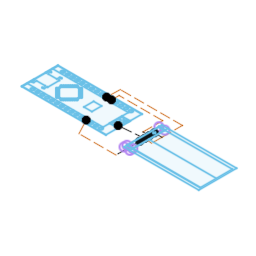
2020_09_18_Arduino & Bluetooth Wood Adaptator V2 v3 (Autodesk Fusion 360 design; units mm, degrees)
Autodesk Fusion 360 part; units mm, degrees
sketch "HC06" plane through (0, 0, 0) normal (0, 0, 1) x (1, 0, 0)
  line L0 (11.524, -5.694) -> (11.524, -4.694)
  line L1 (12.0236, -5.2144) -> (11.0244, -5.2144)
  line L2 (13.0183, 0.206) -> (9.8997, 0.206)
  line L3 (10.024, -1.294) -> (11.524, -1.294)
  circle A0 centre (11.524, -12.694) radius 0.5
  line L4 (10.024, -1.294) -> (11.524, -1.294)
  line L5 (47.724, -17.744) -> (10.024, -17.744)
  line L6 (47.724, -1.294) -> (10.024, -1.294)
  circle A1 centre (11.524, -12.694) radius 0.5
  line L7 (47.724, -9.519) -> (13.024, -9.519)
  line L8 (13.0199, -19.244) -> (48.4034, -19.244)
  line L9 (10.024, -1.294) -> (10.024, 0.206)
  line L10 (48.4034, -19.244) -> (48.4034, 0.206)
  line L11 (13.024, -17.744) -> (13.024, -19.244)
  line L12 (48.4034, 0.206) -> (13.0183, 0.206)
  line L13 (13.024, -1.294) -> (13.024, -17.744)
  line L14 (47.724, -17.744) -> (10.024, -17.744)
  line L15 (13.024, -1.294) -> (13.024, 0.206)
  circle A2 centre (11.524, -5.194) radius 0.5
  line L16 (10.024, -1.294) -> (13.024, -1.294)
  line L17 (47.724, -1.294) -> (47.724, -17.744)
  circle A3 centre (11.524, -5.194) radius 0.5
  line L18 (10.024, -17.744) -> (10.024, -1.294)
  circle A4 centre (11.524, -7.694) radius 0.5
  circle A5 centre (11.524, -7.694) radius 0.5
  line L19 (10.024, -1.294) -> (13.024, -1.294)
  circle A6 centre (11.524, -10.194) radius 0.5
  circle A7 centre (11.524, -10.194) radius 0.5
  line L20 (12.0236, -5.2144) -> (11.0244, -5.2144)
  line L21 (11.524, -5.694) -> (11.524, -4.694)
  line L22 (13.024, -1.294) -> (13.024, -17.744)
  line L23 (13.024, -19.244) -> (10.024, -19.244)
  line L24 (10.024, -17.744) -> (10.024, -1.294)
  line L25 (10.024, -17.744) -> (10.024, -19.244)
sketch "ArduinoNano" plane through (0, 0, 0) normal (0, 0, 1) x (1, 0, 0)
  arc A0 (-42.68, -4.5943) -> (-42.08, -4.5943) centre (-42.38, -4.2943) ccw
  line L0 (0, 0) -> (-43.18, 0)
  line L1 (-42.88, -12.271) -> (-43.18, -12.271)
  line L2 (-36.48, -13.7477) -> (-36.68, -13.9477)
  arc A1 (-36.68, -13.9477) -> (-37.28, -13.9477) centre (-36.98, -14.2477) ccw
  line L3 (-43.18, -6.271) -> (-42.88, -6.271)
  arc A2 (-37.28, -4.5943) -> (-36.68, -4.5943) centre (-36.98, -4.2943) ccw
  line L4 (0, -6.771) -> (0, 0)
  line L5 (-36.68, -4.5943) -> (-36.48, -4.7943)
  line L6 (-43.18, -18.542) -> (0, -18.542)
  line L7 (0, -11.771) -> (0, -6.771)
  arc A3 (-42.88, -13.7477) -> (-42.88, -12.271) centre (-43.6183, -13.0093) ccw
  line L8 (-42.88, -6.271) -> (-42.88, -4.7943)
  line L9 (-36.48, -6.271) -> (-36.18, -6.271)
  line L10 (-42.68, -13.9477) -> (-42.88, -13.7477)
  line L11 (-41.88, -6.271) -> (-37.48, -6.271)
  line L12 (-43.18, 0) -> (-43.18, -6.271)
  line L13 (-37.48, -4.7943) -> (-37.28, -4.5943)
  line L14 (-42.08, -4.5943) -> (-41.88, -4.7943)
  arc A4 (-37.48, -13.7477) -> (-37.48, -12.271) centre (-38.2183, -13.0093) ccw
  line L15 (-42.88, -4.7943) -> (-42.68, -4.5943)
  line L16 (-37.28, -13.9477) -> (-37.48, -13.7477)
  line L17 (-36.48, -12.271) -> (-36.48, -13.7477)
  line L18 (0, -18.542) -> (0, -11.771)
  arc A5 (-36.48, -4.7943) -> (-36.48, -6.271) centre (-35.7416, -5.5326) ccw
  line L19 (-36.18, -12.271) -> (-36.48, -12.271)
  line L20 (-37.48, -12.271) -> (-41.88, -12.271)
  line L21 (-37.48, -6.271) -> (-37.48, -4.7943)
  line L22 (-41.88, -12.271) -> (-41.88, -13.7477)
  line L23 (-36.18, -6.271) -> (-36.18, -12.271)
  arc A6 (-41.88, -4.7943) -> (-41.88, -6.271) centre (-41.1416, -5.5326) ccw
  circle A7 centre (-14.156, -1.524) radius 0.889
  circle A8 centre (-3, -9.271) radius 0.76
  arc A9 (-24.6374, -12.0012) -> (-24.6374, -12.2841) centre (-24.7789, -12.1427) cw
  arc A10 (-31.1356, -5.671) -> (-30.8528, -5.671) centre (-30.9942, -5.8124) cw
  line L24 (-25.3179, -11.9006) -> (-25.028, -11.6107)
  circle A11 centre (-14.156, -17.018) radius 0.889
  circle A12 centre (-3.0017, -7.271) radius 0.76
  line L25 (-18.0694, -11.771) -> (-18.0694, -6.771)
  line L26 (-18.0694, -6.771) -> (-13.9686, -6.771)
  circle A13 centre (-14.156, -17.018) radius 0.5
  circle A14 centre (-24.156, -1.524) radius 0.5
  circle A15 centre (-6.656, -17.018) radius 0.889
  line L27 (0, -6.0786) -> (0, -12.4635)
  circle A16 centre (-19.156, -17.018) radius 0.5
  line L28 (-4.2, -15.829) -> (-4.2, -2.8014)
  line L29 (-13.9686, -6.771) -> (-13.9686, -11.771)
  circle A17 centre (-11.656, -17.018) radius 0.889
  line L30 (-30.8528, -5.671) -> (-30.4622, -6.0616)
  line L31 (-30.7521, -6.3515) -> (-31.1427, -5.9609)
  line L32 (-4.2, -12.4635) -> (-4.2, -6.0786)
  circle A18 centre (-9.156, -1.524) radius 0.889
  circle A19 centre (-16.656, -1.524) radius 0.889
  line L33 (-31.1427, -5.6781) -> (-31.1356, -5.671)
  line L34 (-43.18, 0) -> (-43.18, -18.542)
  arc A20 (-42.08, -13.9477) -> (-42.68, -13.9477) centre (-42.38, -14.2477) ccw
  arc A21 (-31.2001, -12.8065) -> (-31.2001, -12.5236) centre (-31.0587, -12.665) cw
  line L35 (-13.9686, -11.771) -> (-18.0694, -11.771)
  line L36 (0, -12.4635) -> (-4.2, -12.4635)
  circle A22 centre (-9.156, -17.018) radius 0.5
  line L37 (-19.156, -1.524) -> (-19.156, -1.024)
  circle A23 centre (-6.656, -17.018) radius 0.5
  circle A24 centre (-16.656, -17.018) radius 0.889
  circle A25 centre (-19.156, -1.524) radius 0.5
  line L38 (-21.656, -1.524) -> (-21.656, -1.024)
  line L39 (-31.1931, -12.8135) -> (-31.2001, -12.8065)
  circle A26 centre (-6.656, -1.524) radius 0.5
  line L40 (-41.88, -13.7477) -> (-42.08, -13.9477)
  circle A27 centre (-9.156, -17.018) radius 0.889
  line L41 (-0.9965, -7.771) -> (-0.9965, -6.511)
  arc A28 (-24.6445, -12.2912) -> (-24.9274, -12.2912) centre (-24.7859, -12.1497) cw
  line L42 (-24.6374, -12.2841) -> (-24.6445, -12.2912)
  circle A29 centre (-14.156, -1.524) radius 0.5
  line L43 (-24.9274, -12.2912) -> (-25.3179, -11.9006)
  line L44 (-31.2001, -12.5236) -> (-30.8096, -12.133)
  line L45 (-30.4622, -6.0616) -> (-30.7521, -6.3515)
  arc A30 (-31.1427, -5.9609) -> (-31.1427, -5.6781) centre (-31.0013, -5.8195) cw
  line L46 (-19.156, -16.518) -> (-19.156, -17.018)
  circle A31 centre (-9.156, -1.524) radius 0.5
  arc A32 (-30.9102, -12.8135) -> (-31.1931, -12.8135) centre (-31.0517, -12.6721) cw
  line L47 (-24.156, -1.524) -> (-24.156, -1.024)
  line L48 (-12.156, -17.018) -> (-11.156, -17.018)
  circle A33 centre (-11.656, -1.524) radius 0.5
  line L49 (-0.2361, -7.271) -> (-1.7561, -7.271)
  line L50 (-25.028, -11.6107) -> (-24.6374, -12.0012)
  line L51 (-43.18, -12.271) -> (-43.18, -18.542)
  line L52 (-4.2, -6.0786) -> (0, -6.0786)
  circle A34 centre (-4.156, -17.018) radius 0.5
  circle A35 centre (-24.156, -1.524) radius 0.889
  circle A36 centre (-11.656, -17.018) radius 0.5
  circle A37 centre (-16.656, -1.524) radius 0.5
  line L53 (-11.656, -17.518) -> (-11.656, -16.518)
  line L54 (-39.156, -1.524) -> (-39.156, -1.024)
  arc A38 (-27.9093, -14.0003) -> (-28.0507, -14.0589) centre (-28.0507, -13.8589) cw
  arc A39 (-32.9678, -9.1417) -> (-32.9093, -9.0003) centre (-32.7678, -9.1417) cw
  arc A40 (-32.9093, -9.5417) -> (-32.9678, -9.4003) centre (-32.7678, -9.4003) cw
  circle A41 centre (-6.656, -1.524) radius 0.889
  line L55 (-31.3319, -6.9313) -> (-31.7225, -6.5407)
  line L56 (-43.18, -18.542) -> (-43.18, 0)
  line L57 (-28.0507, -14.0589) -> (-28.3093, -14.0589)
  line L58 (-33.1721, -7.9903) -> (-32.7815, -8.3809)
  arc A42 (-23.3921, -9.4003) -> (-23.4507, -9.5417) centre (-23.5921, -9.4003) cw
  circle A43 centre (-16.656, -17.018) radius 0.5
  arc A44 (-31.7225, -6.5407) -> (-31.7225, -6.2579) centre (-31.5811, -6.3993) cw
  line L59 (-31.6218, -7.2212) -> (-31.9118, -7.5112)
  arc A45 (-33.4549, -7.9903) -> (-33.1721, -7.9903) centre (-33.3135, -8.1317) cw
  circle A46 centre (-31.656, -17.018) radius 0.889
  circle A47 centre (-34.156, -1.524) radius 0.5
  line L60 (-31.7225, -6.2579) -> (-31.7154, -6.2508)
  line L61 (-32.3023, -6.8377) -> (-32.2953, -6.8307)
  line L62 (-31.4326, -6.2508) -> (-31.042, -6.6414)
  line L63 (-30.5196, -12.4229) -> (-30.9102, -12.8135)
  line L64 (-30.8096, -12.133) -> (-30.5196, -12.4229)
  line L65 (-34.156, -1.524) -> (-34.156, -1.024)
  circle A48 centre (-3, -11.269) radius 0.76
  line L66 (-33.1359, -8.7353) -> (-33.5265, -8.3447)
  line L67 (-1.0002, -12.0199) -> (-1.0002, -10.4999)
  line L68 (-28.4507, -14.0003) -> (-32.9093, -9.5417)
  circle A49 centre (-0.9961, -7.271) radius 0.76
  circle A50 centre (-36.656, -1.524) radius 0.5
  arc A51 (-28.3093, -14.0589) -> (-28.4507, -14.0003) centre (-28.3093, -13.8589) cw
  line L69 (-32.8822, -7.4176) -> (-32.8751, -7.4105)
  line L70 (-26.4776, -13.0602) -> (-26.1877, -12.7703)
  line L71 (-36.656, -1.524) -> (-36.656, -1.024)
  line L72 (-28.3093, -4.4831) -> (-28.0507, -4.4831)
  line L73 (-26.1877, -12.7703) -> (-25.7971, -13.1609)
  arc A52 (-32.2953, -6.8307) -> (-32.0124, -6.8307) centre (-32.1539, -6.9721) cw
  line L74 (-32.9093, -9.0003) -> (-28.4507, -4.5417)
  line L75 (-26.087, -13.4508) -> (-26.4776, -13.0602)
  arc A53 (-25.8042, -13.4508) -> (-26.087, -13.4508) centre (-25.9456, -13.3094) cw
  circle A54 centre (-36.656, -1.524) radius 0.889
  arc A55 (-32.8751, -7.4105) -> (-32.5923, -7.4105) centre (-32.7337, -7.5519) cw
  arc A56 (-32.3023, -7.1206) -> (-32.3023, -6.8377) centre (-32.1609, -6.9791) cw
  circle A57 centre (-31.656, -1.524) radius 0.5
  arc A58 (-32.8822, -7.7004) -> (-32.8822, -7.4176) centre (-32.7408, -7.559) cw
  circle A59 centre (-4.156, -1.524) radius 0.5
  line L76 (-31.042, -6.6414) -> (-31.3319, -6.9313)
  line L77 (-27.9093, -4.5417) -> (-23.4507, -9.0003)
  line L78 (-23.4507, -9.5417) -> (-27.9093, -14.0003)
  line L79 (-25.7971, -13.4437) -> (-25.8042, -13.4508)
  circle A60 centre (-4.156, -1.524) radius 0.889
  arc A61 (-31.7154, -6.2508) -> (-31.4326, -6.2508) centre (-31.574, -6.3922) cw
  line L80 (-31.9118, -7.5112) -> (-32.3023, -7.1206)
  line L81 (-32.7815, -8.3809) -> (-33.1359, -8.7353)
  line L82 (-32.9678, -9.4003) -> (-32.9678, -9.1417)
  arc A62 (-28.4507, -4.5417) -> (-28.3093, -4.4831) centre (-28.3093, -4.6831) cw
  circle A63 centre (-34.156, -17.018) radius 0.889
  line L83 (-6.656, -17.518) -> (-6.656, -16.518)
  line L84 (-23.3921, -9.1417) -> (-23.3921, -9.4003)
  line L85 (-33.5265, -8.0618) -> (-33.4549, -7.9903)
  arc A64 (-33.5265, -8.3447) -> (-33.5265, -8.0618) centre (-33.385, -8.2033) cw
  arc A65 (-25.7971, -13.1609) -> (-25.7971, -13.4437) centre (-25.9385, -13.3023) cw
  circle A66 centre (-39.156, -1.524) radius 0.889
  circle A67 centre (-1.0002, -11.2599) radius 0.76
  line L86 (-32.0124, -6.8307) -> (-31.6218, -7.2212)
  line L87 (-25.1598, -6.0184) -> (-25.5504, -6.409)
  line L88 (-23.2241, -8.7353) -> (-23.521, -8.4384)
  line L89 (-24.1008, -7.8585) -> (-23.7102, -7.4679)
  arc A68 (-29.976, -4.5113) -> (-29.6931, -4.5113) centre (-29.8345, -4.6528) cw
  line L90 (-32.2017, -7.8011) -> (-32.4916, -8.091)
  line L91 (-25.1669, -5.7285) -> (-25.1598, -5.7355)
  arc A69 (-23.4507, -9.0003) -> (-23.3921, -9.1417) centre (-23.5921, -9.1417) cw
  arc A70 (-25.1598, -5.7355) -> (-25.1598, -6.0184) centre (-25.3012, -5.8769) cw
  line L92 (-29.6931, -4.5113) -> (-29.3025, -4.9019)
  line L93 (-32.4916, -8.091) -> (-32.8822, -7.7004)
  line L94 (-29.3025, -4.9019) -> (-29.5924, -5.1918)
  circle A71 centre (-19.156, -17.018) radius 0.889
  arc A72 (-25.4497, -5.7285) -> (-25.1669, -5.7285) centre (-25.3083, -5.8699) cw
  line L95 (-23.8109, -8.1484) -> (-24.1008, -7.8585)
  line L96 (-24.9706, -6.9888) -> (-25.2605, -6.6989)
  line L97 (-25.8403, -6.119) -> (-25.4497, -5.7285)
  line L98 (-25.7467, -5.1486) -> (-25.7396, -5.1557)
  arc A73 (-24.0002, -6.8952) -> (-24.0002, -7.178) centre (-24.1416, -7.0366) cw
  line L99 (-27, -4.9594) -> (-26.6094, -4.5688)
  arc A74 (-28.0507, -4.4831) -> (-27.9093, -4.5417) centre (-28.0507, -4.6831) cw
  line L100 (-32.5923, -7.4105) -> (-32.2017, -7.8011)
  line L101 (-26.1302, -5.8291) -> (-26.4201, -5.5392)
  arc A75 (-26.0296, -5.1486) -> (-25.7467, -5.1486) centre (-25.8881, -5.2901) cw
  arc A76 (-29.4032, -4.2214) -> (-29.4032, -3.9386) centre (-29.2618, -4.08) cw
  line L102 (-24.0002, -7.178) -> (-24.3907, -7.5686)
  arc A77 (-30.5558, -5.0912) -> (-30.2729, -5.0912) centre (-30.4144, -5.2326) cw
  line L103 (-30.2729, -5.0912) -> (-29.8824, -5.4818)
  arc A78 (-29.3891, -3.9245) -> (-29.1063, -3.9245) centre (-29.2477, -4.0659) cw
  line L104 (-23.4274, -7.4679) -> (-23.4203, -7.475)
  line L105 (-30.1723, -5.7717) -> (-30.5629, -5.3811)
  arc A79 (-26.6094, -4.5688) -> (-26.3265, -4.5688) centre (-26.468, -4.7102) cw
  arc A80 (-27.2537, -3.9245) -> (-26.9708, -3.9245) centre (-27.1122, -4.0659) cw
  arc A81 (-26.3195, -4.5759) -> (-26.3195, -4.8587) centre (-26.4609, -4.7173) cw
  arc A82 (-23.1304, -8.0478) -> (-22.8476, -8.0478) centre (-22.989, -8.1892) cw
  arc A83 (-24.8699, -6.3083) -> (-24.5871, -6.3083) centre (-24.7285, -6.4497) cw
  line L106 (-22.8476, -8.0478) -> (-22.8335, -8.0618)
  line L107 (-23.4203, -7.7579) -> (-23.8109, -8.1484)
  line L108 (-23.521, -8.4384) -> (-23.1304, -8.0478)
  arc A84 (-24.2901, -6.8881) -> (-24.0072, -6.8881) centre (-24.1486, -7.0295) cw
  line L109 (-37.156, -17.018) -> (-36.156, -17.018)
  line L110 (-24.3907, -7.5686) -> (-24.6807, -7.2787)
  line L111 (-24.0072, -6.8881) -> (-24.0002, -6.8952)
  line L112 (-26.4201, -5.5392) -> (-26.0296, -5.1486)
  line L113 (-29.1063, -3.9245) -> (-28.7157, -4.3151)
  line L114 (-30.5629, -5.0982) -> (-30.5558, -5.0912)
  line L115 (-27.2899, -4.6695) -> (-27.6443, -4.3151)
  line L116 (-29.0126, -4.612) -> (-29.4032, -4.2214)
  line L117 (-26.9708, -3.9245) -> (-26.8993, -3.996)
  line L118 (-29.4032, -3.9386) -> (-29.3891, -3.9245)
  line L119 (-26.3195, -4.8587) -> (-26.7101, -5.2493)
  line L120 (-28.7157, -4.3151) -> (-29.0126, -4.612)
  arc A85 (-30.5629, -5.3811) -> (-30.5629, -5.0982) centre (-30.4214, -5.2397) cw
  line L121 (-29.8824, -5.4818) -> (-30.1723, -5.7717)
  line L122 (-25.2605, -6.6989) -> (-24.8699, -6.3083)
  arc A86 (-24.58, -6.3154) -> (-24.58, -6.5982) centre (-24.7214, -6.4568) cw
  line L123 (-22.8335, -8.3447) -> (-23.2241, -8.7353)
  arc A87 (-23.4203, -7.475) -> (-23.4203, -7.7579) centre (-23.5618, -7.6164) cw
  arc A88 (-23.7102, -7.4679) -> (-23.4274, -7.4679) centre (-23.5688, -7.6094) cw
  line L124 (-26.8993, -4.2789) -> (-27.2899, -4.6695)
  line L125 (-24.6807, -7.2787) -> (-24.2901, -6.8881)
  line L126 (-26.3265, -4.5688) -> (-26.3195, -4.5759)
  line L127 (-25.5504, -6.409) -> (-25.8403, -6.119)
  arc A89 (-26.8993, -3.996) -> (-26.8993, -4.2789) centre (-27.0407, -4.1375) cw
  line L128 (-24.5871, -6.3083) -> (-24.58, -6.3154)
  arc A90 (-22.8335, -8.0618) -> (-22.8335, -8.3447) centre (-22.9749, -8.2033) cw
  line L129 (-27.6443, -4.3151) -> (-27.2537, -3.9245)
  line L130 (-32.9326, -11.0741) -> (-32.9396, -11.067)
  line L131 (-29.36, -13.5826) -> (-29.7506, -13.9732)
  line L132 (-26.3769, -14.0236) -> (-26.384, -14.0306)
  arc A91 (-30.6203, -13.3863) -> (-30.6203, -13.1034) centre (-30.4789, -13.2449) cw
  arc A92 (-32.9396, -11.067) -> (-32.9396, -10.7841) centre (-32.7982, -10.9256) cw
  line L133 (-32.9396, -10.7841) -> (-32.549, -10.3935)
  arc A93 (-29.4607, -14.5459) -> (-29.4607, -14.2631) centre (-29.3192, -14.4045) cw
  line L134 (-26.656, -1.524) -> (-26.656, -1.024)
  line L135 (-25.7396, -5.4385) -> (-26.1302, -5.8291)
  line L136 (-30.0405, -13.6833) -> (-29.6499, -13.2927)
  line L137 (-31.9692, -10.9734) -> (-31.6793, -11.2633)
  line L138 (-24.58, -6.5982) -> (-24.9706, -6.9888)
  line L139 (-25.2173, -12.8639) -> (-25.2243, -12.871)
  arc A94 (-25.7396, -5.1557) -> (-25.7396, -5.4385) centre (-25.8811, -5.2971) cw
  line L140 (-29.983, -4.5184) -> (-29.976, -4.5113)
  line L141 (-26.7101, -5.2493) -> (-27, -4.9594)
  arc A95 (-32.3598, -11.6468) -> (-32.3598, -11.364) centre (-32.2184, -11.5054) cw
  line L142 (-32.3598, -11.364) -> (-31.9692, -10.9734)
  arc A96 (-29.983, -4.8013) -> (-29.983, -4.5184) centre (-29.8416, -4.6598) cw
  line L143 (-26.9568, -14.6034) -> (-26.9708, -14.6175)
  line L144 (-30.0334, -13.9732) -> (-30.0405, -13.9661)
  circle A97 centre (-24.156, -17.018) radius 0.5
  circle A98 centre (-26.656, -1.524) radius 0.5
  arc A99 (-26.3769, -13.7407) -> (-26.3769, -14.0236) centre (-26.5183, -13.8822) cw
  line L145 (-29.156, -1.524) -> (-29.156, -1.024)
  line L146 (-29.0701, -13.8725) -> (-28.7157, -14.2269)
  line L147 (-27.2537, -14.6175) -> (-27.6443, -14.2269)
  arc A100 (-26.9708, -14.6175) -> (-27.2537, -14.6175) centre (-27.1122, -14.4761) cw
  circle A101 centre (-29.156, -1.524) radius 0.5
  line L148 (-29.4607, -14.2631) -> (-29.0701, -13.8725)
  arc A102 (-26.384, -14.0306) -> (-26.6668, -14.0306) centre (-26.5254, -13.8892) cw
  line L149 (-31.3894, -11.5532) -> (-31.0995, -11.8431)
  arc A103 (-29.7506, -13.9732) -> (-30.0334, -13.9732) centre (-29.892, -13.8318) cw
  line L150 (-27.0574, -13.6401) -> (-26.7675, -13.3501)
  circle A104 centre (-29.156, -17.018) radius 0.889
  line L151 (-27.6443, -14.2269) -> (-27.3473, -13.93)
  arc A105 (-31.78, -12.2266) -> (-31.78, -11.9438) centre (-31.6386, -12.0852) cw
  circle A106 centre (-24.156, -17.018) radius 0.889
  arc A107 (-30.0405, -13.9661) -> (-30.0405, -13.6833) centre (-29.8991, -13.8247) cw
  line L152 (-30.6132, -13.3934) -> (-30.6203, -13.3863)
  line L153 (-30.6203, -13.1034) -> (-30.2297, -12.7129)
  line L154 (-31.7729, -12.2337) -> (-31.78, -12.2266)
  line L155 (-26.6668, -14.0306) -> (-27.0574, -13.6401)
  line L156 (-31.78, -11.9438) -> (-31.3894, -11.5532)
  line L157 (-31.6793, -11.2633) -> (-32.0699, -11.6539)
  arc A108 (-32.0699, -11.6539) -> (-32.3527, -11.6539) centre (-32.2113, -11.5125) cw
  line L158 (-29.6499, -13.2927) -> (-29.36, -13.5826)
  line L159 (-25.5072, -12.871) -> (-25.8978, -12.4804)
  line L160 (-32.3527, -11.6539) -> (-32.3598, -11.6468)
  line L161 (-25.6079, -12.1905) -> (-25.2173, -12.5811)
  line L162 (-29.3891, -14.6175) -> (-29.4607, -14.5459)
  line L163 (-25.8978, -12.4804) -> (-25.6079, -12.1905)
  arc A109 (-26.9568, -14.3206) -> (-26.9568, -14.6034) centre (-27.0982, -14.462) cw
  line L164 (-30.2297, -12.7129) -> (-29.9398, -13.0028)
  line L165 (-29.5924, -5.1918) -> (-29.983, -4.8013)
  arc A110 (-25.2173, -12.5811) -> (-25.2173, -12.8639) centre (-25.3587, -12.7225) cw
  line L166 (-27.3473, -13.93) -> (-26.9568, -14.3206)
  line L167 (-26.7675, -13.3501) -> (-26.3769, -13.7407)
  line L168 (-28.7157, -14.2269) -> (-29.1063, -14.6175)
  arc A111 (-31.4901, -12.2337) -> (-31.7729, -12.2337) centre (-31.6315, -12.0923) cw
  arc A112 (-29.1063, -14.6175) -> (-29.3891, -14.6175) centre (-29.2477, -14.4761) cw
  circle A113 centre (-29.156, -1.524) radius 0.889
  line L169 (-31.0995, -11.8431) -> (-31.4901, -12.2337)
  line L170 (-29.9398, -13.0028) -> (-30.3304, -13.3934)
  line L171 (-31.656, -1.524) -> (-31.656, -1.024)
  arc A114 (-33.5265, -10.4801) -> (-33.5265, -10.1973) centre (-33.385, -10.3387) cw
  line L172 (-23.5785, -10.1611) -> (-23.2241, -9.8067)
  line L173 (-24.156, -16.518) -> (-24.156, -17.018)
  arc A115 (-24.0576, -11.4214) -> (-24.0576, -11.7043) centre (-24.199, -11.5628) cw
  line L174 (-24.3475, -11.7113) -> (-24.7381, -11.3207)
  circle A116 centre (-26.656, -1.524) radius 0.889
  line L175 (-32.549, -10.3935) -> (-32.2591, -10.6835)
  line L176 (-29.156, -16.518) -> (-29.156, -17.018)
  line L177 (-23.7677, -11.1315) -> (-24.1583, -10.7409)
  line L178 (-32.839, -10.1036) -> (-33.2295, -10.4942)
  line L179 (-24.1583, -10.7409) -> (-23.8684, -10.451)
  circle A117 centre (-29.156, -17.018) radius 0.5
  line L180 (-32.2591, -10.6835) -> (-32.6497, -11.0741)
  arc A118 (-25.2243, -12.871) -> (-25.5072, -12.871) centre (-25.3658, -12.7296) cw
  line L181 (-21.656, -16.518) -> (-21.656, -17.018)
  circle A119 centre (-39.156, -17.018) radius 0.889
  arc A120 (-33.2295, -10.4942) -> (-33.5124, -10.4942) centre (-33.371, -10.3528) cw
  line L182 (-33.5265, -10.1973) -> (-33.1359, -9.8067)
  line L183 (-33.5124, -10.4942) -> (-33.5265, -10.4801)
  circle A121 centre (-26.656, -17.018) radius 0.889
  arc A122 (-32.6497, -11.0741) -> (-32.9326, -11.0741) centre (-32.7911, -10.9326) cw
  circle A123 centre (-19.156, -1.524) radius 0.889
  arc A124 (-23.4778, -10.8416) -> (-23.4778, -11.1244) centre (-23.6192, -10.983) cw
  line L184 (-23.8684, -10.451) -> (-23.4778, -10.8416)
  arc A125 (-30.3304, -13.3934) -> (-30.6132, -13.3934) centre (-30.4718, -13.2519) cw
  circle A126 centre (-21.656, -1.524) radius 0.5
  line L185 (0, -18.542) -> (-43.18, -18.542)
  line L186 (-22.8335, -10.4801) -> (-22.905, -10.5517)
  circle A127 centre (-26.656, -17.018) radius 0.5
  arc A128 (-22.8335, -10.1973) -> (-22.8335, -10.4801) centre (-22.9749, -10.3387) cw
  circle A129 centre (-31.656, -17.018) radius 0.5
  line L187 (-16.656, -16.518) -> (-16.656, -17.018)
  circle A130 centre (-34.156, -1.524) radius 0.9737
  line L188 (-4.2, -2.8014) -> (-43.18, -2.8014)
  line L189 (-23.1879, -10.5517) -> (-23.5785, -10.1611)
  circle A131 centre (-31.656, -1.524) radius 0.9737
  circle A132 centre (-36.656, -17.018) radius 0.889
  arc A133 (-22.905, -10.5517) -> (-23.1879, -10.5517) centre (-23.0465, -10.4103) cw
  line L190 (-23.4778, -11.1244) -> (-23.4849, -11.1315)
  arc A134 (-24.0647, -11.7113) -> (-24.3475, -11.7113) centre (-24.2061, -11.5699) cw
  line L191 (-26.656, -16.518) -> (-26.656, -17.018)
  line L192 (-24.0576, -11.7043) -> (-24.0647, -11.7113)
  circle A135 centre (-39.156, -17.018) radius 0.5
  arc A136 (-23.4849, -11.1315) -> (-23.7677, -11.1315) centre (-23.6263, -10.9901) cw
  circle A137 centre (-39.156, -1.524) radius 0.5
  line L193 (-36.656, -17.518) -> (-36.656, -16.518)
  line L194 (-24.4482, -11.0308) -> (-24.0576, -11.4214)
  line L195 (-24.7381, -11.3207) -> (-24.4482, -11.0308)
  circle A138 centre (-36.656, -17.018) radius 0.5
  circle A139 centre (-21.656, -17.018) radius 0.889
  line L196 (-33.1359, -9.8067) -> (-32.839, -10.1036)
  circle A140 centre (-21.656, -17.018) radius 0.5
  line L197 (-4.2, -15.829) -> (-43.18, -15.829)
  circle A141 centre (-0.998, -9.271) radius 0.76
  line L198 (-11.656, -2.024) -> (-11.656, -1.024)
  circle A142 centre (-4.156, -17.018) radius 0.889
  circle A143 centre (-34.156, -17.018) radius 0.5
  line L199 (-14.156, -16.518) -> (-14.156, -17.018)
  line L200 (-43.18, 0) -> (0, 0)
  line L201 (-23.2241, -9.8067) -> (-22.8335, -10.1973)
  circle A144 centre (-11.656, -1.524) radius 0.889
  circle A145 centre (-21.656, -1.524) radius 0.889
sketch "Join Arduino to HC06" plane through (0, 0, 0) normal (0, 0, 1) x (1, 0, 0)
  circle A0 centre (-6.656, -17.018) radius 0.889
  circle A1 centre (-11.656, -17.018) radius 0.889
  circle A2 centre (-14.156, -1.524) radius 0.889
  circle A3 centre (-16.656, -1.524) radius 0.889
  line L0 (-11.656, -17.518) -> (-11.656, -16.518) construction
  line L1 (-11.656, -17.018) -> (-11.656, -17.518) construction
  line L2 (47.724, -9.519) -> (13.024, -9.519) construction
  line L3 (0, -18.542) -> (-43.18, -18.542) construction
  line L4 (13.024, -17.744) -> (13.024, -1.294) construction
  line L5 (11.524, -7.694) -> (15.524, -7.694) construction
  line L6 (11.524, -5.194) -> (18.524, -5.194) construction
  line L7 (18.524, -5.194) -> (18.524, -24.1605) construction
  line L8 (-6.656, -17.018) -> (-6.656, -18.542) construction
  line L9 (-6.656, -18.542) -> (-6.656, -22.542) construction
  line L10 (-11.656, -17.018) -> (-11.656, -18.542) construction
  line L11 (-11.656, -18.542) -> (-11.656, -25.542) construction
  line L12 (-11.656, -25.542) -> (18.524, -25.542) construction
  line L13 (18.524, -25.542) -> (18.524, -24.1605)
  line L14 (-6.656, -22.542) -> (15.524, -22.542) construction
  line L15 (15.524, -22.542) -> (15.524, -7.694) construction
  line L16 (-43.18, 0) -> (0, 0)
  line L17 (-16.656, -1.524) -> (-16.656, 0) construction
  line L18 (-16.656, 0) -> (-16.656, -1.9072) construction
  line L19 (-16.656, -1.9072) -> (-16.656, 5.0928) construction
  line L20 (10.024, -17.744) -> (10.024, -1.294)
  line L21 (11.524, -10.194) -> (10.024, -10.194) construction
  line L22 (10.024, -10.194) -> (7.024, -10.194) construction
  line L23 (7.024, -10.194) -> (7.024, 5.0928) construction
  line L24 (7.024, 5.0928) -> (-16.656, 5.0928) construction
  line L25 (-14.156, -1.524) -> (-14.156, 2.476) construction
  line L26 (0, -6.771) -> (0, 0)
  line L27 (0, 0) -> (4, 0) construction
  line L28 (-14.156, 2.476) -> (-13.3035, 2.476)
  line L29 (-13.3035, 2.476) -> (4, 2.476) construction
  line L30 (11.524, -12.694) -> (4, -12.694) construction
  line L31 (4, -12.694) -> (4, 0) construction
  line L32 (4, -22.542) -> (4, -12.694) construction
  line L33 (5.25, -2.847) -> (2.75, -2.847)
  line L34 (2.75, -2.847) -> (2.75, -9.847)
  line L35 (2.75, -9.847) -> (5.25, -9.847)
  line L36 (5.25, -9.847) -> (5.25, -2.847)
  line L37 (5.25, -2.847) -> (2.75, -9.847) construction
  line L38 (2.75, -2.847) -> (5.25, -9.847) construction
  line L39 (5.25, -14.118) -> (2.75, -14.118)
  line L40 (2.75, -14.118) -> (2.75, -21.118)
  line L41 (2.75, -21.118) -> (5.25, -21.118)
  line L42 (5.25, -21.118) -> (5.25, -14.118)
  line L43 (5.25, -14.118) -> (2.75, -21.118) construction
  line L44 (2.75, -14.118) -> (5.25, -21.118) construction
  line L45 (-15.901, -1.524) -> (-15.901, 5.0928)
  arc A4 (-15.901, 5.0928) -> (-17.411, 5.0928) centre (-16.656, 5.0928) ccw
  line L46 (-17.411, 5.0928) -> (-17.411, -1.524)
  arc A5 (-17.411, -1.524) -> (-15.901, -1.524) centre (-16.656, -1.524) ccw
  line L47 (-16.656, -1.524) -> (-16.656, 5.0928) construction
  line L48 (-16.656, 4.3378) -> (7.024, 4.3378)
  arc A6 (7.024, 4.3378) -> (7.024, 5.8478) centre (7.024, 5.0928) ccw
  line L49 (7.024, 5.8478) -> (-16.656, 5.8478)
  arc A7 (-16.656, 5.8478) -> (-16.656, 4.3378) centre (-16.656, 5.0928) ccw
  line L50 (-16.656, 5.0928) -> (7.024, 5.0928) construction
  line L51 (6.269, 5.0928) -> (6.269, -10.194)
  arc A8 (6.269, -10.194) -> (7.779, -10.194) centre (7.024, -10.194) ccw
  line L52 (7.779, -10.194) -> (7.779, 5.0928)
  arc A9 (7.779, 5.0928) -> (6.269, 5.0928) centre (7.024, 5.0928) ccw
  line L53 (7.024, 5.0928) -> (7.024, -10.194) construction
  line L54 (7.024, -10.949) -> (11.524, -10.949)
  arc A10 (11.524, -10.949) -> (11.524, -9.439) centre (11.524, -10.194) ccw
  line L55 (11.524, -9.439) -> (7.024, -9.439)
  arc A11 (7.024, -9.439) -> (7.024, -10.949) centre (7.024, -10.194) ccw
  line L56 (7.024, -10.194) -> (11.524, -10.194) construction
  line L57 (11.524, -5.949) -> (18.524, -5.949)
  arc A12 (18.524, -5.949) -> (18.524, -4.439) centre (18.524, -5.194) ccw
  line L58 (18.524, -4.439) -> (11.524, -4.439)
  arc A13 (11.524, -4.439) -> (11.524, -5.949) centre (11.524, -5.194) ccw
  line L59 (11.524, -5.194) -> (18.524, -5.194) construction
  line L60 (11.524, -8.449) -> (15.524, -8.449)
  arc A14 (15.524, -8.449) -> (15.524, -6.939) centre (15.524, -7.694) ccw
  line L61 (15.524, -6.939) -> (11.524, -6.939)
  arc A15 (11.524, -6.939) -> (11.524, -8.449) centre (11.524, -7.694) ccw
  line L62 (11.524, -7.694) -> (15.524, -7.694) construction
  line L63 (14.769, -7.694) -> (14.769, -22.542)
  arc A16 (14.769, -22.542) -> (16.279, -22.542) centre (15.524, -22.542) ccw
  line L64 (16.279, -22.542) -> (16.279, -7.694)
  arc A17 (16.279, -7.694) -> (14.769, -7.694) centre (15.524, -7.694) ccw
  line L65 (15.524, -7.694) -> (15.524, -22.542) construction
  line L66 (17.769, -5.194) -> (17.769, -25.542)
  arc A18 (17.769, -25.542) -> (19.279, -25.542) centre (18.524, -25.542) ccw
  line L67 (19.279, -25.542) -> (19.279, -5.194)
  arc A19 (19.279, -5.194) -> (17.769, -5.194) centre (18.524, -5.194) ccw
  line L68 (18.524, -5.194) -> (18.524, -25.542) construction
  line L69 (15.524, -21.787) -> (-6.656, -21.787)
  arc A20 (-6.656, -21.787) -> (-6.656, -23.297) centre (-6.656, -22.542) ccw
  line L70 (-6.656, -23.297) -> (15.524, -23.297)
  arc A21 (15.524, -23.297) -> (15.524, -21.787) centre (15.524, -22.542) ccw
  line L71 (15.524, -22.542) -> (-6.656, -22.542) construction
  line L72 (-5.901, -22.542) -> (-5.901, -17.018)
  arc A22 (-5.901, -17.018) -> (-7.411, -17.018) centre (-6.656, -17.018) ccw
  line L73 (-7.411, -17.018) -> (-7.411, -22.542)
  arc A23 (-7.411, -22.542) -> (-5.901, -22.542) centre (-6.656, -22.542) ccw
  line L74 (-6.656, -22.542) -> (-6.656, -17.018) construction
  line L75 (18.524, -24.787) -> (-11.656, -24.787)
  arc A24 (-11.656, -24.787) -> (-11.656, -26.297) centre (-11.656, -25.542) ccw
  line L76 (-11.656, -26.297) -> (18.524, -26.297)
  arc A25 (18.524, -26.297) -> (18.524, -24.787) centre (18.524, -25.542) ccw
  line L77 (18.524, -25.542) -> (-11.656, -25.542) construction
  line L78 (-10.901, -25.542) -> (-10.901, -17.018)
  arc A26 (-10.901, -17.018) -> (-12.411, -17.018) centre (-11.656, -17.018) ccw
  line L79 (-12.411, -17.018) -> (-12.411, -25.542)
  arc A27 (-12.411, -25.542) -> (-10.901, -25.542) centre (-11.656, -25.542) ccw
  line L80 (-11.656, -25.542) -> (-11.656, -17.018) construction
  line L81 (4.755, -22.542) -> (4.755, 2.476)
  arc A28 (4.755, 2.476) -> (3.245, 2.476) centre (4, 2.476) ccw
  line L82 (3.245, 2.476) -> (3.245, -22.542)
  arc A29 (3.245, -22.542) -> (4.755, -22.542) centre (4, -22.542) ccw
  line L83 (4, -22.542) -> (4, 2.476) construction
  line L84 (11.524, -11.939) -> (4, -11.939)
  arc A30 (4, -11.939) -> (4, -13.449) centre (4, -12.694) ccw
  line L85 (4, -13.449) -> (11.524, -13.449)
  arc A31 (11.524, -13.449) -> (11.524, -11.939) centre (11.524, -12.694) ccw
  line L86 (11.524, -12.694) -> (4, -12.694) construction
  line L87 (4, 3.231) -> (-14.156, 3.231)
  arc A32 (-14.156, 3.231) -> (-14.156, 1.721) centre (-14.156, 2.476) ccw
  line L88 (-14.156, 1.721) -> (4, 1.721)
  arc A33 (4, 1.721) -> (4, 3.231) centre (4, 2.476) ccw
  line L89 (4, 2.476) -> (-14.156, 2.476) construction
  line L90 (-14.911, 2.476) -> (-14.911, -1.524)
  arc A34 (-14.911, -1.524) -> (-13.401, -1.524) centre (-14.156, -1.524) ccw
  line L91 (-13.401, -1.524) -> (-13.401, 2.476)
  arc A35 (-13.401, 2.476) -> (-14.911, 2.476) centre (-14.156, 2.476) ccw
  line L92 (-14.156, 2.476) -> (-14.156, -1.524) construction
  line L93 (0, -11.771) -> (0, -6.771)
  line L94 (-1.0002, -11.2599) -> (1.4998, -11.2599) construction
  circle A36 centre (-1.0002, -11.2599) radius 0.755
  circle A37 centre (1.4998, -11.2599) radius 1.2
  circle A38 centre (-4.156, -17.018) radius 0.755
  circle A39 centre (-2.7685, -19.9379) radius 1.2
  circle A40 centre (11.524, -10.194) radius 0.755
  circle A41 centre (11.524, -12.694) radius 0.755
  circle A42 centre (11.524, -7.694) radius 0.755
  circle A43 centre (11.524, -5.194) radius 0.755
  line L95 (11.524, -5.194) -> (10.024, -5.194) construction
  line L96 (10.024, -5.194) -> (9.024, -5.194) construction
  line L97 (10.024, -7.694) -> (9.024, -7.694) construction
  circle A44 centre (9.024, -5.194) radius 0.755
  circle A45 centre (9.024, -7.694) radius 0.755
  line L98 (9.024, -5.949) -> (11.524, -5.949)
  arc A46 (11.524, -5.949) -> (11.524, -4.439) centre (11.524, -5.194) ccw
  line L99 (11.524, -4.439) -> (9.024, -4.439)
  arc A47 (9.024, -4.439) -> (9.024, -5.949) centre (9.024, -5.194) ccw
  line L100 (9.024, -5.194) -> (11.524, -5.194) construction
  line L101 (9.024, -8.449) -> (11.524, -8.449)
  arc A48 (11.524, -8.449) -> (11.524, -6.939) centre (11.524, -7.694) ccw
  line L102 (11.524, -6.939) -> (9.024, -6.939)
  arc A49 (9.024, -6.939) -> (9.024, -8.449) centre (9.024, -7.694) ccw
  line L103 (9.024, -7.694) -> (11.524, -7.694) construction
  point P0 (-6.656, -17.018)
  point P1 (-11.656, -17.018)
  point P2 (-14.156, -1.524)
  point P3 (-16.656, -1.524)
  point P4 (-11.656, -17.518)
  point P5 (11.524, -7.694)
  point P6 (11.524, -5.194)
  point P7 (11.524, -10.194)
  point P8 (11.524, -12.694)
  point P9 (4, -12.694)
  point P10 (4, -22.542)
  point P11 (4, -6.347)
  point P12 (4, -17.618)
  point P13 (-1.0002, -11.2599)
  point P14 (-4.156, -17.018)
  dimension "d1" = 4
  dimension "d2" = 7
  dimension "d3" = 4
  dimension "d4" = 7
  dimension "d5" = 7
  dimension "d6" = 3
  dimension "d7" = 4
  dimension "d8" = 4
  dimension "d9" = 2.5
  dimension "d10" = 7
  dimension "d11" = 2.5
  dimension "d12" = 7
  dimension "d15" = 1.51
  dimension "d16" = 1.51
  dimension "d17" = 1.51
  dimension "d18" = 1.51
  dimension "d19" = 1.51
  dimension "d20" = 1.51
  dimension "d21" = 1.51
  dimension "d22" = 1.51
  dimension "d23" = 1.51
  dimension "d24" = 1.51
  dimension "d25" = 1.51
  dimension "d26" = 1.51
  dimension "d27" = 1.51
  dimension "d28" = 1.51
  dimension "d29" = 1.51
  dimension "d30" = 1.51
  dimension "d34" = 2.5
  dimension "d36" = 1.51
  dimension "d37" = 2.4
  dimension "d38" = 1.51
  dimension "d39" = 2.4
  dimension "d42" = 1.51
  dimension "d43" = 1.51
  dimension "d44" = 1.51
  dimension "d45" = 1.51
  dimension "d46" = 1
  dimension "d47" = 1
  dimension "d48" = 1.51
  dimension "d49" = 1.51
  dimension "d50" = 1.51
  dimension "d51" = 1.51
  constraint coincident P0 A0.centre
  constraint coincident P1 A1.centre
  constraint coincident P2 A2.centre
  constraint coincident P3 A3.centre
  constraint coincident P4 L0.start
  constraint coincident P5 L5.start
  constraint coincident P6 L6.start
  constraint perpendicular L4 L6
  constraint coincident L3 L8.end
  constraint perpendicular L3 L8
  constraint perpendicular L3 L9
  constraint coincident L3 L10.end
  constraint perpendicular L3 L10
  constraint perpendicular L3 L11
  constraint perpendicular L7 L12
  constraint perpendicular L12 L13
  constraint perpendicular L7 L14
  constraint perpendicular L5 L15
  constraint coincident L16 L17.end
  constraint perpendicular L6 L17
  constraint perpendicular L16 L18
  constraint perpendicular L16 L19
  constraint coincident P7 L21.start
  constraint coincident L20 L21.end
  constraint perpendicular L20 L21
  constraint perpendicular L20 L22
  constraint perpendicular L22 L23
  constraint perpendicular L19 L24
  constraint perpendicular L16 L25
  constraint coincident L16.end L26.end
  constraint perpendicular L26 L27
  constraint perpendicular L25 L28
  constraint perpendicular L25 L29
  constraint coincident P8 L30.start
  constraint coincident P9 L30.end
  constraint perpendicular L27 L31
  constraint coincident P10 L32.start
  constraint perpendicular L30 L32
  constraint horizontal L33
  constraint perpendicular L33 L34
  constraint parallel L33 L35
  constraint parallel L34 L36
  constraint coincident L37 P11
  constraint coincident L38 P11
  constraint midpoint L31 P11
  constraint horizontal L39
  constraint perpendicular L39 L40
  constraint parallel L39 L41
  constraint parallel L40 L42
  constraint coincident L43 P12
  constraint coincident L44 P12
  constraint midpoint L32 P12
  constraint tangent L45 A4
  constraint tangent A4 L46
  constraint parallel L45 L46
  constraint tangent L46 A5
  constraint tangent L45 A5
  constraint perpendicular L24 L47
  constraint tangent L48 A6
  constraint tangent A6 L49
  constraint parallel L48 L49
  constraint tangent L49 A7
  constraint tangent L48 A7
  constraint coincident L23.end L24.start
  constraint perpendicular L23 L50
  constraint coincident L19.end L24.end
  constraint tangent L51 A8
  constraint tangent A8 L52
  constraint parallel L51 L52
  constraint tangent L52 A9
  constraint tangent L51 A9
  constraint coincident L22.end L23.start
  constraint perpendicular L22 L53
  constraint tangent L54 A10
  constraint tangent A10 L55
  constraint parallel L54 L55
  constraint tangent L55 A11
  constraint tangent L54 A11
  constraint perpendicular L20 L56
  constraint tangent L57 A12
  constraint tangent A12 L58
  constraint parallel L57 L58
  constraint tangent L58 A13
  constraint tangent L57 A13
  constraint coincident L6.end L7.start
  constraint perpendicular L7 L59
  constraint tangent L60 A14
  constraint tangent A14 L61
  constraint parallel L60 L61
  constraint tangent L61 A15
  constraint tangent L60 A15
  constraint coincident L5.end L15.end
  constraint perpendicular L15 L62
  constraint tangent L63 A16
  constraint tangent A16 L64
  constraint parallel L63 L64
  constraint tangent L64 A17
  constraint tangent L63 A17
  constraint coincident L14.end L15.start
  constraint perpendicular L14 L65
  constraint tangent L66 A18
  constraint tangent A18 L67
  constraint parallel L66 L67
  constraint tangent L67 A19
  constraint tangent L66 A19
  constraint coincident L12.end L13.start
  constraint perpendicular L12 L68
  constraint tangent L69 A20
  constraint tangent A20 L70
  constraint parallel L69 L70
  constraint tangent L70 A21
  constraint tangent L69 A21
  constraint coincident L9.end L14.start
  constraint perpendicular L9 L71
  constraint tangent L72 A22
  constraint tangent A22 L73
  constraint parallel L72 L73
  constraint tangent L73 A23
  constraint tangent L72 A23
  constraint perpendicular L71 L74
  constraint tangent L75 A24
  constraint tangent A24 L76
  constraint parallel L75 L76
  constraint tangent L76 A25
  constraint tangent L75 A25
  constraint coincident L11.end L12.start
  constraint perpendicular L11 L77
  constraint tangent L78 A26
  constraint tangent A26 L79
  constraint parallel L78 L79
  constraint tangent L79 A27
  constraint tangent L78 A27
  constraint tangent L81 A28
  constraint tangent A28 L82
  constraint parallel L81 L82
  constraint tangent L82 A29
  constraint tangent L81 A29
  constraint coincident L29.end A28.centre
  constraint perpendicular L29 L83
  constraint tangent L84 A30
  constraint tangent A30 L85
  constraint parallel L84 L85
  constraint tangent L85 A31
  constraint tangent L84 A31
  constraint perpendicular L31 L86
  constraint tangent L87 A32
  constraint tangent A32 L88
  constraint parallel L87 L88
  constraint tangent L88 A33
  constraint tangent L87 A33
  constraint coincident L25.end L28.start
  constraint perpendicular L25 L89
  constraint tangent L90 A34
  constraint tangent A34 L91
  constraint parallel L90 L91
  constraint tangent L91 A35
  constraint tangent L90 A35
  constraint perpendicular L16 L92
  constraint coincident P13 L94.start
  constraint perpendicular L93 L94
  constraint coincident L94.end A37.centre
  constraint coincident P14 A38.centre
  constraint concentric A13 A43
  constraint coincident L20 L95.end
  constraint perpendicular L20 L95
  constraint perpendicular L20 L96
  constraint coincident L20 L97.start
  constraint perpendicular L20 L97
  constraint coincident L96.end A44.centre
  constraint coincident L97.end A45.centre
  constraint tangent L98 A46
  constraint tangent A46 L99
  constraint parallel L98 L99
  constraint tangent L99 A47
  constraint tangent L98 A47
  constraint tangent L101 A48
  constraint tangent A48 L102
  constraint parallel L101 L102
  constraint tangent L102 A49
  constraint tangent L101 A49
  constraint parallel L62 L103
  measures "d1" distance of P5 L5.end
  measures "d2" distance of P6 L6.end
  measures "d3" distance of L8.end L9.end
  measures "d4" distance of L10.end L11.end
  measures "d5" distance of L18.end L19.end
  measures "d6" distance of L21.end L22.end
  measures "d7" distance of P2 L25.end
  measures "d8" distance of L16.end L27.end
  measures "d9" distance of L34.end L35.end
  measures "d10" distance of L33.end L34.end
  measures "d11" distance of L40.end L41.end
  measures "d12" distance of L39.end L40.end
  measures "d15" diameter of A4
  measures "d16" diameter of A6
  measures "d17" diameter of A8
  measures "d18" diameter of A10
  measures "d19" diameter of A12
  measures "d20" diameter of A14
  measures "d21" diameter of A16
  measures "d22" diameter of A18
  measures "d23" diameter of A20
  measures "d24" diameter of A22
  measures "d25" diameter of A24
  measures "d26" diameter of A26
  measures "d27" diameter of A28
  measures "d28" diameter of A30
  measures "d29" diameter of A32
  measures "d30" diameter of A34
  measures "d34" distance of P13 L94.end
  measures "d36" diameter of A36
  measures "d37" diameter of A37
  measures "d38" diameter of A38
  measures "d39" diameter of A39
  measures "d42" diameter of A40
  measures "d43" diameter of A41
  measures "d44" diameter of A42
  measures "d45" diameter of A43
  measures "d46" distance of L95.end L96.end
  measures "d47" distance of L97.start L97.end
  measures "d48" diameter of A44
  measures "d49" diameter of A45
  measures "d50" diameter of A46
  measures "d51" diameter of A48
sketch "CutAround" plane through (0, 0, 0) normal (0, 0, 1) x (1, 0, 0)
  line L0 (-44.1103, 12.8228) -> (50.9491, 12.8228)
  line L1 (50.9491, 12.8228) -> (50.9491, -34.251)
  line L2 (50.9491, -34.251) -> (-44.1103, -34.251)
  line L3 (-44.1103, -34.251) -> (-44.1103, 12.8228)
  constraint horizontal L0
  constraint vertical L1
  constraint horizontal L2
  constraint vertical L3
extrude "Extrude1" add sketch "CutAround" against normal blind 17 makes body 1
extrude "Extrude2" cut sketch "Join Arduino to HC06" against normal blind 17 contours A0 L72 A22 L73 | L69 A20 L72 A23 | L81 L84 A30 L85 | A15 A42 A48 | A45 A49 | A31 A41 | A10 A40 | A8 L52 L55 A11 | A32 L88 L91 A35 | L45 A4 L48 A7 | A1 L78 A26 L79 | L75 A24 L78 A27 | A13 A43 A46 | A44 A47 | A36 | A37 | A38 | A39 picked at (-6.656, -17.3143) picked at (-11.656, -17.3143) bodies 1
extrude "Extrude3" add sketch "Join Arduino to HC06" against normal blind 2.5 separate body contours A0 L72 A22 L73 | A0 L69 A20 L72 L73 | L69 A20 L72 A23 | L69 L70 L72 A23 L82 A29 | L41 L69 L81 L82 | L69 L81 L82 A29 | L63 A16 L69 L70 L81 A29 | L39 L41 L81 L82 | L39 L40 L41 L82 | L63 A16 L69 A21 | L60 A14 L63 L64 L69 A21 | L39 L41 L42 L81 | L39 L81 L82 A30 L85 | L60 A14 L63 A17 | L60 L61 L63 A17 A42 A48 | L35 L81 L82 L84 A30 | L81 L84 A30 L85 | L20 A15 A42 L101 L102 | A15 A42 A48 | L20 L81 L84 L85 | L33 L35 L81 L82 | L33 L34 L35 L82 | L20 A45 L101 L102 | L20 L84 L85 A41 | L33 L35 L36 L81 | L33 L81 L82 L88 A33 | L20 L54 L55 A40 | L20 A8 L52 L54 L55 | A45 A49 | A31 A41 | A28 L82 L87 L88 L91 A35 | A28 L82 L88 A33 | A10 A40 | L48 A6 L51 L52 L55 A11 | A8 L52 L55 A11 | L16 A32 L88 L90 L91 | A32 L88 L91 A35 | L48 A6 L51 A9 | A2 L16 L90 L91 | L45 A4 L48 L49 L51 A9 | A2 L90 A34 L91 | L45 A4 L48 A7 | A3 L16 L45 L46 | L16 L45 L46 L48 A7 | A3 L45 L46 A5 | A1 L78 A26 L79 | A1 L75 A24 L78 L79 | L75 A24 L78 A27 | L66 A18 L75 L76 L78 A27 | L66 A18 L75 A25 | L57 A12 L66 L67 L75 A25 | L57 A12 L66 A19 | L57 L58 L66 A19 A43 A46 | L20 A13 A43 L98 L99 | A13 A43 A46 | L20 A44 L98 L99 | A44 A47 picked at (-6.656, -17.3143) picked at (-14.156, -1.2277) picked at (-16.656, -1.2277) picked at (-11.656, -17.3143) makes body 2 at (-1.121, 5.3444, 0) makes body 3 at (8.2123, -25.7937, 0) makes body 4 at (4.541, -22.7937, 0)
combine "Combine1" operation cut target body 1 tool bodies 2 3 4
sketch "VerticalHC06Base" plane through (0, 0, 0) normal (0, 0, 1) x (1, 0, 0)
  line L0 (10.024, -1.294) -> (13.024, -1.294)
  line L1 (13.024, -17.744) -> (10.024, -17.744)
  line L2 (11.524, -1.294) -> (11.524, -17.744) construction
  line L3 (12.574, -1.294) -> (10.474, -1.294)
  line L4 (10.474, -1.294) -> (10.474, -17.744)
  line L5 (10.474, -17.744) -> (12.574, -17.744)
  line L6 (12.574, -17.744) -> (12.574, -1.294)
  line L7 (12.574, -1.294) -> (10.474, -17.744) construction
  line L8 (10.474, -1.294) -> (12.574, -17.744) construction
  line L9 (12.574, -1.294) -> (15.074, -1.294)
  line L10 (15.074, -1.294) -> (15.074, -17.744)
  line L11 (15.074, -17.744) -> (12.574, -17.744)
  line L12 (12.574, -17.744) -> (12.574, -1.294)
  point P0 (11.524, -9.519)
  point P1 (11.524, -9.519)
  dimension "d60" = 2.1
  dimension "d61" = 2.5
  dimension "d62" = 16.45
  constraint midpoint L0 L2.start
  constraint midpoint L1 L2.end
  constraint coincident L2 P1
  constraint midpoint L2 P1
  constraint horizontal L3
  constraint perpendicular L3 L4
  constraint parallel L3 L5
  constraint parallel L4 L6
  constraint coincident L7 P1
  constraint coincident L8 P1
  constraint coincident P1 P0
  constraint horizontal L9
  constraint vertical L10
  constraint horizontal L11
  constraint vertical L12
  measures "d60" distance of L4.end L5.end
  measures "d61" distance of L3.start L9.end
  measures "d62" distance of L3.start L5.end
extrude "Extrude7" add sketch "VerticalHC06Base" against normal blind 2.8 separate body contours L0 L1 L3 L4 L5 L6 L12 makes body 5
combine "Combine3" operation cut target body 1 tool bodies 5
sketch "Sketch6" plane through (0, 0, 0) normal (0, 0, 1) x (1, 0, 0)
  line L0 (13.024, -19.244) -> (10.024, -19.244) construction
  line L1 (11.524, -12.694) -> (11.524, -24.9142) construction
  line L2 (11.524, -24.9142) -> (-7.4525, -24.9142) construction
  line L3 (-7.4525, -24.9142) -> (-11.656, -17.018) construction
  line L4 (13.024, -1.294) -> (13.024, -17.744) construction
  line L5 (11.524, -5.194) -> (15.4505, -5.194) construction
  line L6 (15.4505, -5.194) -> (15.4505, -10.5097) construction
  line L7 (15.4505, -10.5097) -> (11.524, -10.194) construction
  line L8 (11.524, -10.194) -> (-1.0002, -11.2599) construction
  line L9 (15.4505, -5.194) -> (15.4505, 5.3157) construction
  line L10 (15.4505, 5.3157) -> (-16.4667, 5.3157) construction
  line L11 (-16.4667, 5.3157) -> (-16.656, -1.524) construction
  line L12 (10.024, -17.744) -> (10.024, -1.294) construction
  line L13 (11.524, -7.694) -> (8.2192, -7.694) construction
  line L14 (8.2192, -7.694) -> (8.2192, 2.3797) construction
  line L15 (8.2192, 2.3797) -> (-14.1299, 2.3797) construction
  line L16 (-14.1299, 2.3797) -> (-14.156, -1.524) construction
  point P0 (11.524, -12.694)
  point P1 (-11.656, -17.018)
  point P2 (11.524, -5.194)
  point P3 (11.524, -10.194)
  point P4 (-1.0002, -11.2599)
  point P5 (-16.656, -1.524)
  point P6 (11.524, -7.694)
  point P7 (-14.156, -1.524)
  constraint coincident P0 L1.start
  constraint perpendicular L0 L1
  constraint perpendicular L1 L2
  constraint coincident P1 L3.end
  constraint coincident P2 L5.start
  constraint perpendicular L4 L5
  constraint perpendicular L5 L6
  constraint coincident P3 L7.end
  constraint coincident P4 L8.end
  constraint perpendicular L5 L9
  constraint perpendicular L6 L10
  constraint coincident P5 L11.end
  constraint coincident P6 L13.start
  constraint perpendicular L12 L13
  constraint perpendicular L5 L14
  constraint perpendicular L12 L15
  constraint coincident P7 L16.end
hidden bodies 1
equation "HorizontalTunnelSize = 1.51 mm"
equation "VerticalTunnelSize = 2.4 mm"
equation "d15 = HorizontalTunnelSize"
equation "d16 = HorizontalTunnelSize"
equation "d17 = HorizontalTunnelSize"
equation "d18 = HorizontalTunnelSize"
equation "d19 = HorizontalTunnelSize"
equation "d20 = HorizontalTunnelSize"
equation "d21 = HorizontalTunnelSize"
equation "d22 = HorizontalTunnelSize"
equation "d23 = HorizontalTunnelSize"
equation "d24 = HorizontalTunnelSize"
equation "d25 = HorizontalTunnelSize"
equation "d26 = HorizontalTunnelSize"
equation "d27 = HorizontalTunnelSize"
equation "d28 = HorizontalTunnelSize"
equation "d29 = HorizontalTunnelSize"
equation "d30 = HorizontalTunnelSize"
equation "WoodHeight = 17 mm"
equation "d32 = -WoodHeight"
equation "CableJoinHoleSize = 1.51 mm"
equation "d36 = CableJoinHoleSize"
equation "d37 = VerticalTunnelSize"
equation "d38 = CableJoinHoleSize"
equation "d39 = VerticalTunnelSize"
equation "d40 = -WoodHeight"
equation "d42 = CableJoinHoleSize"
equation "d43 = CableJoinHoleSize"
equation "d44 = CableJoinHoleSize"
equation "d45 = CableJoinHoleSize"
equation "d48 = CableJoinHoleSize"
equation "d49 = CableJoinHoleSize"
equation "d50 = CableJoinHoleSize"
equation "d51 = CableJoinHoleSize"
named bodies: "WoodBoard", "HC06Hole"
